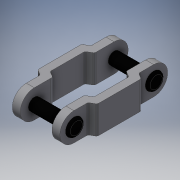
# Autodesk Inventor part: Connector_1
Saved by Autodesk Inventor 2018.1 (Build 221151000, 151)
## iProperties
Created: 2012-05-30
Part Number: Connector_1
Material: Generic
Document SubType Name: Modeling
Designer: normanpa
Density: 1 g/cm^3
Appearance: Default
Author: normanpa
Autodesk Inventor part; units mm, degrees
ref_plane "YZ Plane" through (0, 0, 0) normal (1, 0, 0) x (0, 1, 0)
ref_plane "XZ Plane" through (0, 0, 0) normal (0, 1, 0) x (-1, 0, 0)
ref_plane "XY Plane" through (0, 0, 0) normal (0, 0, 1) x (1, 0, 0)
sketch "Sketch1" plane through (0, 0, 0) normal (0, 1, 0) x (-1, 0, 0)
  line L0 (-9.4742, 21.4376) -> (-6.3, 21.4376)
  line L1 (-9.4742, 21.4376) -> (-9.4742, 10.8898)
  line L2 (-9.9742, 10.0237) -> (-11.3618, 9.2226)
  arc A0 (-11.3618, 9.2226) -> (-11.8618, 8.3566) centre (-10.8618, 8.3566) ccw
  arc A1 (-9.9742, 10.0237) -> (-9.4742, 10.8898) centre (-10.4742, 10.8898) ccw
  line L3 (-11.8618, 8.3566) -> (-11.8618, -7.902)
  arc A2 (-11.8618, -7.902) -> (-11.3618, -8.768) centre (-10.8618, -7.902) ccw
  line L4 (-11.3618, -8.768) -> (-9.9742, -9.5691)
  arc A3 (-9.4742, -10.4351) -> (-9.9742, -9.5691) centre (-10.4742, -10.4351) ccw
  line L5 (-9.4742, -10.4351) -> (-9.4742, -21.4376)
  line L6 (-9.4742, -21.4376) -> (-6.2738, -21.4376)
  line L7 (-6.2738, -21.4376) -> (-6.2738, -8.7047)
  arc A4 (-6.2738, -8.7047) -> (-6.7738, -7.8387) centre (-7.2738, -8.7047) ccw
  line L8 (-6.7738, -7.8387) -> (-8.263, -6.9789)
  arc A5 (-8.763, -6.1129) -> (-8.263, -6.9789) centre (-7.763, -6.1129) ccw
  line L9 (-8.763, -6.1129) -> (-8.763, 6.5675)
  arc A6 (-8.263, 7.4335) -> (-8.763, 6.5675) centre (-7.763, 6.5675) ccw
  line L10 (-8.263, 7.4335) -> (-6.7738, 8.2933)
  arc A7 (-6.7738, 8.2933) -> (-6.3, 9.3867) centre (-7.2738, 9.1593) ccw
  line L11 (-6.3, 9.3867) -> (-6.3, 21.4376)
  line L12 (0, 0) -> (0, 4.0406) construction
  line L13 (9.4742, 21.4376) -> (6.3, 21.4376)
  line L14 (9.4742, 21.4376) -> (9.4742, 10.8898)
  line L15 (9.9742, 10.0237) -> (11.3618, 9.2226)
  arc A8 (11.8618, 8.3566) -> (11.3618, 9.2226) centre (10.8618, 8.3566) ccw
  arc A9 (9.4742, 10.8898) -> (9.9742, 10.0237) centre (10.4742, 10.8898) ccw
  line L16 (11.8618, 8.3566) -> (11.8618, -7.902)
  arc A10 (11.3618, -8.768) -> (11.8618, -7.902) centre (10.8618, -7.902) ccw
  line L17 (11.3618, -8.768) -> (9.9742, -9.5691)
  arc A11 (9.9742, -9.5691) -> (9.4742, -10.4351) centre (10.4742, -10.4351) ccw
  line L18 (9.4742, -10.4351) -> (9.4742, -21.4376)
  line L19 (9.4742, -21.4376) -> (6.2738, -21.4376)
  line L20 (6.2738, -21.4376) -> (6.2738, -8.7047)
  arc A12 (6.7738, -7.8387) -> (6.2738, -8.7047) centre (7.2738, -8.7047) ccw
  line L21 (6.7738, -7.8387) -> (8.263, -6.9789)
  arc A13 (8.263, -6.9789) -> (8.763, -6.1129) centre (7.763, -6.1129) ccw
  line L22 (8.763, -6.1129) -> (8.763, 6.5675)
  arc A14 (8.763, 6.5675) -> (8.263, 7.4335) centre (7.763, 6.5675) ccw
  line L23 (8.263, 7.4335) -> (6.7738, 8.2933)
  arc A15 (6.3, 9.3867) -> (6.7738, 8.2933) centre (7.2738, 9.1593) ccw
  line L24 (6.3, 9.3867) -> (6.3, 21.4376)
  dimension "d21" = 6.3
  dimension "d22" = 12.6
  constraints: 50 end point, 32 point on circle, 28 symmetric about line, 16 centre point, 16 tangent, 9 parallel, 7 equal radius, 1 horizontal, 1 vertical, 8 other
  measures "d21" horizontal distance of L0.end L12.start
  measures "d22" distance between parallel lines of L24 L11
extrude "Extrusion1" add sketch "Sketch1" along normal mid plane 11.1252
full round fillet "Fillet1" first side at (-10.8289, -5.5626, 2.3407) centre faces at (-7.3406, -1.8542, -21.4376) second side at (-10.8289, 5.5626, 2.3407)
full round fillet "Fillet2" first side at (10.8289, -5.5626, 2.3407) centre faces at (7.3406, -1.8542, -21.4376) second side at (10.8289, 5.5626, 2.3407)
full round fillet "Fillet3" first side at (10.8289, 5.5626, 2.3407) centre faces at (7.3581, 1.8542, 21.4376) second side at (10.8289, -5.5626, 2.3407)
full round fillet "Fillet4" first side at (-10.8289, -5.5626, 2.3407) centre faces at (-8.4161, -1.8542, 21.4376) second side at (-10.8289, 5.5626, 2.3407)
hole "Hole1" at (9.4742, 0, -15.875) direction (-1, 0, 0) diameter 4.8006 end through all
hole "Hole2" at (9.4742, 0, 15.875) direction (-1, 0, 0) diameter 4.8006 end through all
sketch "Sketch2" plane through (0, 0, 0) normal (0, 1, 0) x (-1, 0, 0)
  arc A0 (-9.4742, 19.2753) -> (-10.4742, 18.2753) centre (-9.4742, 18.2753) ccw
  line L0 (-10.4742, 15.875) -> (-10.4742, 18.2753)
  arc A1 (10.4742, 18.2753) -> (9.4742, 19.2753) centre (9.4742, 18.2753) ccw
  line L1 (10.4742, 15.875) -> (10.4742, 18.2753)
  line L2 (-9.4742, 18.2753) -> (9.4742, 18.2753)
  line L3 (-10.4742, 15.875) -> (10.4742, 15.875)
  line L4 (-9.4742, 19.2753) -> (-9.4742, 18.2753)
  line L5 (9.4742, 19.2753) -> (9.4742, 18.2753)
  point P0 (0, 0)
  constraints: 12 end point, 4 point on circle, 2 centre point, 1 parallel, 1 perpendicular
revolve "Revolution1" add sketch "Sketch2" angle 360 about axis through (10.4742, 0, 15.875) along (-1, 0, 0) separate body
mirror "Mirror1" about plane through (0, 0, 0) normal (0, 0, 1) of "Revolution1" bodies 2
body "Solid2"
body "Solid3"
